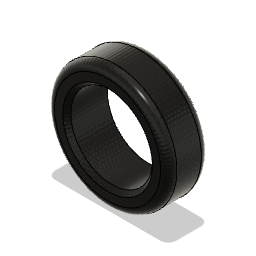
safety_ring (Autodesk Fusion 360 design; units mm, degrees)
Autodesk Fusion 360 part; units mm, degrees
sketch "Esquisse1" plane through (0, 0, 0) normal (0, 0, 1) x (1, 0, 0)
  circle A0 centre (0, 0) radius 10
  circle A1 centre (0, 0) radius 15
  dimension "d1" = 20
  dimension "d2" = 30
  constraint coincident A0.centre A1.centre
  measures "d1" diameter of A0
  measures "d2" diameter of A1
extrude "Extrusion1" add sketch "Esquisse1" along normal blind 10
fillet "Congé1" radius 2 2 edges at (-13.9849, -5.4242, 10) (-13.9849, -5.4242, 0)
chamfer "Chanfrein1" distance 1 angle 45 1 edges at (-9.3233, 3.6162, 10)
